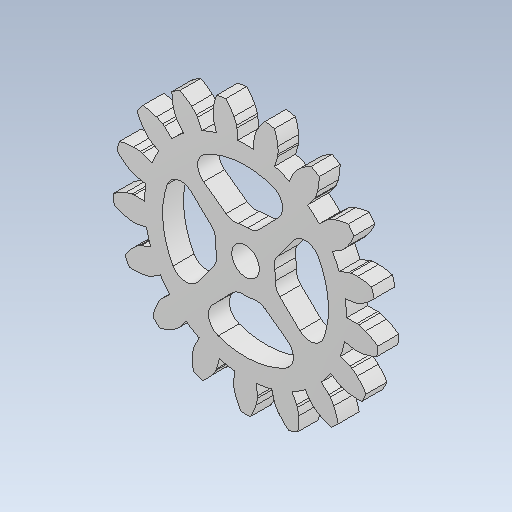
# Autodesk Inventor part: ｍ2歯数17ギアd3.99
Saved by Autodesk Inventor 2020.2 (Build 242310000, 310)
## iProperties
Created: 2020-03-11
Part Number: ｍ2歯数17ギアd3.99
Material: アルミニウム 2014-T4
Document SubType Name: Modeling
Designer: aoyam
Density: 2.8 g/cm^3
Appearance: サテン
Mass: 7.2939 g
Surface Area: 24.4586 cm^2
Volume: 2.60496 cm^3
Author: aoyam
Autodesk Inventor part; units mm, degrees
ref_plane "YZ Plane" through (0, 0, 0) normal (1, 0, 0) x (0, 1, 0)
ref_plane "XZ Plane" through (0, 0, 0) normal (0, 1, 0) x (-1, 0, 0)
ref_plane "XY Plane" through (0, 0, 0) normal (0, 0, 1) x (1, 0, 0)
sketch "スケッチ1" plane through (0, 0, 0) normal (0, 0, 1) x (1, 0, 0)
  arc A0 (3.6531, 18.9504) -> (3.5922, 18.6594) centre (5.3094, 18.4521) ccw
  arc A1 (4.0246, 19.8629) -> (3.6531, 18.9504) centre (8.2422, 17.6137) ccw
  arc A2 (5.1821, 21.5212) -> (4.0246, 19.8629) centre (11.4021, 15.9465) ccw
  arc A3 (1.1187, 18.6594) -> (1.0579, 18.9504) centre (-0.5985, 18.4521) ccw
  arc A4 (1.0579, 18.9504) -> (0.6864, 19.8629) centre (-3.5313, 17.6137) ccw
  arc A5 (0.6864, 19.8629) -> (-0.4711, 21.5212) centre (-6.6912, 15.9465) ccw
  arc A6 (3.478, 17.1891) -> (1.2329, 17.1891) centre (2.3555, 2.7326) ccw
  arc A7 (-0.4711, 21.5212) -> (-1.796, 21.2735) centre (2.3555, 2.7326) ccw
  line L0 (3.478, 17.1891) -> (3.5922, 18.6594)
  line L1 (1.2329, 17.1891) -> (1.1187, 18.6594)
  arc A8 (-4.5512, 17.1371) -> (-4.7131, 17.3865) centre (-6.0775, 16.3235) ccw
  line L2 (-3.9136, 15.8073) -> (-4.5512, 17.1371)
  arc A9 (-1.8201, 16.6184) -> (-3.9136, 15.8073) centre (2.3555, 2.7326) ccw
  line L3 (-1.8201, 16.6184) -> (-2.2447, 18.0307)
  arc A10 (-2.2931, 18.324) -> (-2.2447, 18.0307) centre (-0.5686, 18.4577) ccw
  arc A11 (-2.2763, 19.3091) -> (-2.2931, 18.324) centre (2.469, 18.7354) ccw
  arc A12 (-1.796, 21.2735) -> (-2.2763, 19.3091) centre (6.0178, 18.3222) ccw
  arc A13 (-4.7131, 17.3865) -> (-5.3891, 18.1031) centre (-8.5095, 14.4823) ccw
  arc A14 (-5.3891, 18.1031) -> (-7.0674, 19.2313) centre (-10.8537, 11.7862) ccw
  arc A15 (-7.0674, 19.2313) -> (-8.2134, 18.5218) centre (2.3555, 2.7326) ccw
  arc A16 (-9.2883, 13.6695) -> (-9.5294, 13.8435) centre (-10.4177, 12.3594) ccw
  line L4 (-8.2134, 12.6598) -> (-9.2883, 13.6695)
  arc A17 (-6.5542, 14.1723) -> (-8.2134, 12.6598) centre (2.3555, 2.7326) ccw
  line L5 (-6.5542, 14.1723) -> (-7.4604, 15.3358)
  arc A18 (-7.6115, 15.5919) -> (-7.4604, 15.3358) centre (-6.0517, 16.3395) ccw
  arc A19 (-7.9516, 16.5165) -> (-7.6115, 15.5919) centre (-3.3195, 17.6958) ccw
  arc A20 (-8.2134, 18.5218) -> (-7.9516, 16.5165) centre (0.1389, 18.5925) ccw
  arc A21 (-9.5294, 13.8435) -> (-10.4186, 14.2675) centre (-12.0203, 9.764) ccw
  arc A22 (-10.4186, 14.2675) -> (-12.3912, 14.7132) centre (-13.2323, 6.4031) ccw
  arc A23 (-12.3912, 14.7132) -> (-13.2034, 13.6376) centre (2.3555, 2.7326) ccw
  arc A24 (-12.4529, 8.7247) -> (-12.7406, 8.7999) centre (-13.0328, 7.0951) ccw
  line L6 (-11.0858, 8.1715) -> (-12.4529, 8.7247)
  arc A25 (-10.0851, 10.1813) -> (-11.0858, 8.1715) centre (2.3555, 2.7326) ccw
  line L7 (-10.0851, 10.1813) -> (-11.3504, 10.9389)
  arc A26 (-11.5838, 11.1231) -> (-11.3504, 10.9389) centre (-10.3994, 12.3836) ccw
  arc A27 (-12.2349, 11.8623) -> (-11.5838, 11.1231) centre (-8.3416, 14.6353) ccw
  arc A28 (-13.2034, 13.6376) -> (-12.2349, 11.8623) centre (-5.4407, 16.7208) ccw
  arc A29 (-12.7406, 8.7999) -> (-13.7229, 8.8741) centre (-13.5896, 4.0961) ccw
  arc A30 (-13.7229, 8.8741) -> (-15.7233, 8.5771) centre (-13.5056, 0.5243) ccw
  arc A31 (-15.7233, 8.5771) -> (-16.0921, 7.2807) centre (2.3555, 2.7326) ccw
  arc A32 (-13.6175, 2.9707) -> (-13.9129, 2.9369) centre (-13.5696, 1.2417) ccw
  line L8 (-12.1429, 2.9487) -> (-13.6175, 2.9707)
  arc A33 (-11.9358, 5.1842) -> (-12.1429, 2.9487) centre (2.3555, 2.7326) ccw
  line L9 (-11.9358, 5.1842) -> (-13.3893, 5.4336)
  arc A34 (-13.6735, 5.521) -> (-13.3893, 5.4336) centre (-13.0244, 7.1243) ccw
  arc A35 (-14.5477, 5.9752) -> (-13.6735, 5.521) centre (-11.9191, 9.9673) ccw
  arc A36 (-16.0921, 7.2807) -> (-14.5477, 5.9752) centre (-9.9674, 12.9599) ccw
  arc A37 (-13.9129, 2.9369) -> (-14.8558, 2.6512) centre (-13.0054, -1.756) ccw
  arc A38 (-14.8558, 2.6512) -> (-16.6138, 1.6516) centre (-11.6368, -5.0563) ccw
  arc A39 (-16.6138, 1.6516) -> (-16.4894, 0.3095) centre (2.3555, 2.7326) ccw
  arc A40 (-12.6249, -2.8155) -> (-12.8882, -2.9537) centre (-11.9556, -4.4104) ccw
  line L10 (-11.2419, -2.3033) -> (-12.6249, -2.8155)
  arc A41 (-11.8563, -0.1439) -> (-11.2419, -2.3033) centre (2.3555, 2.7326) ccw
  line L11 (-11.8563, -0.1439) -> (-13.3018, -0.4365)
  arc A42 (-13.5984, -0.4576) -> (-13.3018, -0.4365) centre (-13.5724, 1.2719) ccw
  arc A43 (-14.5777, -0.3499) -> (-13.5984, -0.4576) centre (-13.5686, 4.3222) ccw
  arc A44 (-16.4894, 0.3095) -> (-14.5777, -0.3499) centre (-12.8297, 7.8177) ccw
  arc A45 (-12.8882, -2.9537) -> (-13.6641, -3.5607) centre (-10.3466, -7.0019) ccw
  arc A46 (-13.6641, -3.5607) -> (-14.9423, -5.1278) centre (-7.8783, -9.5849) ccw
  arc A47 (-14.9423, -5.1278) -> (-14.3415, -6.3344) centre (2.3555, 2.7326) ccw
  arc A48 (-9.6091, -7.8524) -> (-9.8047, -8.0764) centre (-8.4088, -9.0978) ccw
  line L12 (-8.5046, -6.8752) -> (-9.6091, -7.8524)
  arc A49 (-9.8575, -5.0836) -> (-8.5046, -6.8752) centre (2.3555, 2.7326) ccw
  line L13 (-9.8575, -5.0836) -> (-11.0997, -5.8785)
  arc A50 (-11.3686, -6.0054) -> (-11.0997, -5.8785) centre (-11.9691, -4.3833) ccw
  arc A51 (-12.3207, -6.2587) -> (-11.3686, -6.0054) centre (-13.0675, -1.5376) ccw
  arc A52 (-14.3415, -6.3344) -> (-12.3207, -6.2587) centre (-13.6413, 1.9888) ccw
  arc A53 (-9.8047, -8.0764) -> (-10.3089, -8.9227) centre (-5.9724, -10.9331) ccw
  arc A54 (-10.3089, -8.9227) -> (-10.9347, -10.8457) centre (-2.7376, -12.45) ccw
  arc A55 (-10.9347, -10.8457) -> (-9.9386, -11.7538) centre (2.3555, 2.7326) ccw
  arc A56 (-4.9774, -11.4597) -> (-5.0789, -11.7392) centre (-3.4083, -12.1875) ccw
  line L14 (-4.3005, -10.1495) -> (-4.9774, -11.4597)
  arc A57 (-6.2093, -8.9676) -> (-4.3005, -10.1495) centre (2.3555, 2.7326) ccw
  line L15 (-6.2093, -8.9676) -> (-7.0804, -10.1576)
  arc A58 (-7.2854, -10.373) -> (-7.0804, -10.1576) centre (-8.4313, -9.0774) ccw
  arc A59 (-8.0816, -10.9532) -> (-7.2854, -10.373) centre (-10.4835, -6.8207) ccw
  arc A60 (-9.9386, -11.7538) -> (-8.0816, -10.9532) centre (-12.2924, -3.7397) ccw
  arc A61 (-5.0789, -11.7392) -> (-5.2433, -12.7106) centre (-0.4734, -13.0186) ccw
  arc A62 (-5.2433, -12.7106) -> (-5.1322, -14.7298) centre (3.0909, -13.2646) ccw
  arc A63 (-5.1322, -14.7298) -> (-3.8754, -15.2167) centre (2.3555, 2.7326) ccw
  arc A64 (0.6446, -13.1503) -> (0.651, -13.4476) centre (2.3707, -13.2621) ccw
  line L16 (0.8025, -11.684) -> (0.6446, -13.1503)
  arc A65 (-1.4043, -11.2715) -> (0.8025, -11.684) centre (2.3555, 2.7326) ccw
  line L17 (-1.4043, -11.2715) -> (-1.7867, -12.6958)
  arc A66 (-1.9001, -12.9707) -> (-1.7867, -12.6958) centre (-3.4366, -12.1765) ccw
  arc A67 (-2.4329, -13.7993) -> (-1.9001, -12.9707) centre (-6.1655, -10.8135) ccw
  arc A68 (-3.8754, -15.2167) -> (-2.4329, -13.7993) centre (-8.9652, -8.594) ccw
  arc A69 (0.651, -13.4476) -> (0.8485, -14.4127) centre (5.4076, -12.9769) ccw
  arc A70 (0.8485, -14.4127) -> (1.6815, -16.2555) centre (8.8201, -11.9187) ccw
  arc A71 (1.6815, -16.2555) -> (3.0294, -16.2555) centre (2.3555, 2.7326) ccw
  arc A72 (6.4977, -12.6958) -> (6.611, -12.9707) centre (8.1476, -12.1765) ccw
  line L18 (6.1153, -11.2715) -> (6.4977, -12.6958)
  arc A73 (3.9084, -11.684) -> (6.1153, -11.2715) centre (2.3555, 2.7326) ccw
  line L19 (3.9084, -11.684) -> (4.0663, -13.1503)
  arc A74 (4.06, -13.4476) -> (4.0663, -13.1503) centre (2.3403, -13.2621) ccw
  arc A75 (3.8625, -14.4127) -> (4.06, -13.4476) centre (-0.6966, -12.9769) ccw
  arc A76 (3.0294, -16.2555) -> (3.8625, -14.4127) centre (-4.1091, -11.9187) ccw
  arc A77 (6.611, -12.9707) -> (7.1439, -13.7993) centre (10.8764, -10.8135) ccw
  arc A78 (7.1439, -13.7993) -> (8.5863, -15.2167) centre (13.6762, -8.594) ccw
  arc A79 (8.5863, -15.2167) -> (9.8432, -14.7298) centre (2.3555, 2.7326) ccw
  arc A80 (11.7914, -10.1576) -> (11.9963, -10.373) centre (13.1422, -9.0774) ccw
  line L20 (10.9203, -8.9676) -> (11.7914, -10.1576)
  arc A81 (9.0114, -10.1495) -> (10.9203, -8.9676) centre (2.3555, 2.7326) ccw
  line L21 (9.0114, -10.1495) -> (9.6884, -11.4597)
  arc A82 (9.7898, -11.7392) -> (9.6884, -11.4597) centre (8.1193, -12.1875) ccw
  arc A83 (9.9543, -12.7106) -> (9.7898, -11.7392) centre (5.1844, -13.0186) ccw
  arc A84 (9.8432, -14.7298) -> (9.9543, -12.7106) centre (1.6201, -13.2646) ccw
  arc A85 (11.9963, -10.373) -> (12.7925, -10.9532) centre (15.1944, -6.8207) ccw
  arc A86 (12.7925, -10.9532) -> (14.6496, -11.7538) centre (17.0033, -3.7397) ccw
  arc A87 (14.6496, -11.7538) -> (15.6457, -10.8457) centre (2.3555, 2.7326) ccw
  arc A88 (15.8107, -5.8785) -> (16.0796, -6.0054) centre (16.6801, -4.3833) ccw
  line L22 (14.5685, -5.0836) -> (15.8107, -5.8785)
  arc A89 (13.2155, -6.8752) -> (14.5685, -5.0836) centre (2.3555, 2.7326) ccw
  line L23 (13.2155, -6.8752) -> (14.3201, -7.8524)
  arc A90 (14.5156, -8.0764) -> (14.3201, -7.8524) centre (13.1198, -9.0978) ccw
  arc A91 (15.0199, -8.9227) -> (14.5156, -8.0764) centre (10.6833, -10.9331) ccw
  arc A92 (15.6457, -10.8457) -> (15.0199, -8.9227) centre (7.4486, -12.45) ccw
  arc A93 (16.0796, -6.0054) -> (17.0316, -6.2587) centre (17.7785, -1.5376) ccw
  arc A94 (17.0316, -6.2587) -> (19.0525, -6.3344) centre (18.3522, 1.9888) ccw
  arc A95 (19.0525, -6.3344) -> (19.6533, -5.1278) centre (2.3555, 2.7326) ccw
  arc A96 (18.0128, -0.4365) -> (18.3093, -0.4576) centre (18.2833, 1.2719) ccw
  line L24 (16.5673, -0.1439) -> (18.0128, -0.4365)
  arc A97 (15.9529, -2.3033) -> (16.5673, -0.1439) centre (2.3555, 2.7326) ccw
  line L25 (15.9529, -2.3033) -> (17.3359, -2.8155)
  arc A98 (17.5991, -2.9537) -> (17.3359, -2.8155) centre (16.6665, -4.4104) ccw
  arc A99 (18.3751, -3.5607) -> (17.5991, -2.9537) centre (15.0576, -7.0019) ccw
  arc A100 (19.6533, -5.1278) -> (18.3751, -3.5607) centre (12.5892, -9.5849) ccw
  arc A101 (18.3093, -0.4576) -> (19.2886, -0.3499) centre (18.2795, 4.3222) ccw
  arc A102 (19.2886, -0.3499) -> (21.2003, 0.3095) centre (17.5407, 7.8177) ccw
  arc A103 (21.2003, 0.3095) -> (21.3247, 1.6516) centre (2.3555, 2.7326) ccw
  arc A104 (18.1003, 5.4336) -> (18.3844, 5.521) centre (17.7354, 7.1243) ccw
  line L26 (16.6467, 5.1842) -> (18.1003, 5.4336)
  arc A105 (16.8539, 2.9487) -> (16.6467, 5.1842) centre (2.3555, 2.7326) ccw
  line L27 (16.8539, 2.9487) -> (18.3285, 2.9707)
  arc A106 (18.6239, 2.9369) -> (18.3285, 2.9707) centre (18.2805, 1.2417) ccw
  arc A107 (19.5667, 2.6512) -> (18.6239, 2.9369) centre (17.7163, -1.756) ccw
  arc A108 (21.3247, 1.6516) -> (19.5667, 2.6512) centre (16.3477, -5.0563) ccw
  arc A109 (18.3844, 5.521) -> (19.2587, 5.9752) centre (16.63, 9.9673) ccw
  arc A110 (19.2587, 5.9752) -> (20.8031, 7.2807) centre (14.6783, 12.9599) ccw
  arc A111 (20.8031, 7.2807) -> (20.4342, 8.5771) centre (2.3555, 2.7326) ccw
  arc A112 (16.0613, 10.9389) -> (16.2947, 11.1231) centre (15.1103, 12.3836) ccw
  line L28 (14.796, 10.1813) -> (16.0613, 10.9389)
  arc A113 (15.7968, 8.1715) -> (14.796, 10.1813) centre (2.3555, 2.7326) ccw
  line L29 (15.7968, 8.1715) -> (17.1638, 8.7247)
  arc A114 (17.4515, 8.7999) -> (17.1638, 8.7247) centre (17.7437, 7.0951) ccw
  arc A115 (18.4339, 8.8741) -> (17.4515, 8.7999) centre (18.3005, 4.0961) ccw
  arc A116 (20.4342, 8.5771) -> (18.4339, 8.8741) centre (18.2165, 0.5243) ccw
  arc A117 (16.2947, 11.1231) -> (16.9459, 11.8623) centre (13.0526, 14.6353) ccw
  arc A118 (16.9459, 11.8623) -> (17.9144, 13.6376) centre (10.1516, 16.7208) ccw
  arc A119 (17.9144, 13.6376) -> (17.1021, 14.7132) centre (2.3555, 2.7326) ccw
  arc A120 (12.1714, 15.3358) -> (12.3224, 15.5919) centre (10.7627, 16.3395) ccw
  line L30 (11.2652, 14.1723) -> (12.1714, 15.3358)
  arc A121 (12.9243, 12.6598) -> (11.2652, 14.1723) centre (2.3555, 2.7326) ccw
  line L31 (12.9243, 12.6598) -> (13.9993, 13.6695)
  arc A122 (14.2403, 13.8435) -> (13.9993, 13.6695) centre (15.1286, 12.3594) ccw
  arc A123 (15.1296, 14.2675) -> (14.2403, 13.8435) centre (16.7312, 9.764) ccw
  arc A124 (17.1021, 14.7132) -> (15.1296, 14.2675) centre (17.9432, 6.4031) ccw
  arc A125 (12.3224, 15.5919) -> (12.6626, 16.5165) centre (8.0305, 17.6958) ccw
  arc A126 (12.6626, 16.5165) -> (12.9244, 18.5218) centre (4.5721, 18.5925) ccw
  arc A127 (12.9244, 18.5218) -> (11.7784, 19.2313) centre (2.3555, 2.7326) ccw
  arc A128 (6.9557, 18.0307) -> (7.0041, 18.324) centre (5.2796, 18.4577) ccw
  line L32 (6.531, 16.6184) -> (6.9557, 18.0307)
  arc A129 (8.6245, 15.8073) -> (6.531, 16.6184) centre (2.3555, 2.7326) ccw
  line L33 (8.6245, 15.8073) -> (9.2621, 17.1371)
  arc A130 (9.424, 17.3865) -> (9.2621, 17.1371) centre (10.7885, 16.3235) ccw
  arc A131 (10.1001, 18.1031) -> (9.424, 17.3865) centre (13.2204, 14.4823) ccw
  arc A132 (11.7784, 19.2313) -> (10.1001, 18.1031) centre (15.5647, 11.7862) ccw
  arc A133 (7.0041, 18.324) -> (6.9872, 19.3091) centre (2.2419, 18.7354) ccw
  arc A134 (6.9872, 19.3091) -> (6.507, 21.2735) centre (-1.3069, 18.3222) ccw
  arc A135 (6.507, 21.2735) -> (5.1821, 21.5212) centre (2.3555, 2.7326) ccw
  circle A136 centre (2.3555, 2.7326) radius 1.995
  circle A137 centre (2.3555, 2.7326) radius 14.5
  circle A138 centre (2.3555, 2.7326) radius 11.9
  circle A139 centre (2.3555, 2.7326) radius 4.295
  line L34 (2.3555, 2.7326) -> (10.0109, 11.8433)
  line L35 (10.8895, 11.026) -> (6.2096, 4.628)
  line L36 (9.0544, 12.5679) -> (3.5584, 6.8557)
  line L37 (-7.4799, 9.4315) -> (-1.7676, 3.9355)
  line L38 (-5.9379, 11.2666) -> (0.4601, 6.5867)
  line L39 (-4.3435, -7.1028) -> (1.1525, -1.3905)
  line L40 (-6.1786, -5.5608) -> (-1.4987, 0.8372)
  line L41 (12.1908, -3.9664) -> (6.4786, 1.5296)
  line L42 (10.6488, -5.8015) -> (4.2508, -1.1216)
  point P0 (0, 0)
  point P1 (-4.5512, 17.1371)
  point P2 (-4.7131, 17.3865)
  point P3 (-5.3891, 18.1031)
  point P4 (-7.0674, 19.2313)
  point P5 (-8.2134, 18.5218)
  point P6 (-7.9516, 16.5165)
  point P7 (-7.6115, 15.5919)
  point P8 (-7.4604, 15.3358)
  point P9 (-6.5542, 14.1723)
  point P10 (-9.5294, 13.8435)
  point P11 (-10.4186, 14.2675)
  point P12 (-12.3912, 14.7132)
  point P13 (-13.2034, 13.6376)
  point P14 (-11.5838, 11.1231)
  point P15 (-11.3504, 10.9389)
  point P16 (-10.0851, 10.1813)
  point P17 (-11.0858, 8.1715)
  point P18 (-12.4529, 8.7247)
  point P19 (-12.7406, 8.7999)
  point P20 (-13.7229, 8.8741)
  point P21 (-15.7233, 8.5771)
  point P22 (-16.0921, 7.2807)
  point P23 (-14.5477, 5.9752)
  point P24 (-13.6735, 5.521)
  point P25 (-13.3893, 5.4336)
  point P26 (-11.9358, 5.1842)
  point P27 (-12.1429, 2.9487)
  point P28 (-13.6175, 2.9707)
  point P29 (-13.9129, 2.9369)
  point P30 (-14.8558, 2.6512)
  point P31 (-16.6138, 1.6516)
  point P32 (-16.4894, 0.3095)
  point P33 (-14.5777, -0.3499)
  point P34 (-13.5984, -0.4576)
  point P35 (-12.8882, -2.9537)
  point P36 (-13.6641, -3.5607)
  point P37 (-14.9423, -5.1278)
  point P38 (-14.3415, -6.3344)
  point P39 (-12.3207, -6.2587)
  point P40 (-11.3686, -6.0054)
  point P41 (-11.0997, -5.8785)
  point P42 (-9.8575, -5.0836)
  point P43 (-10.3089, -8.9227)
  point P44 (-10.9347, -10.8457)
  point P45 (-9.9386, -11.7538)
  point P46 (-8.0816, -10.9532)
  point P47 (-7.2854, -10.373)
  point P48 (-7.0804, -10.1576)
  point P49 (-5.0789, -11.7392)
  point P50 (-5.2433, -12.7106)
  point P51 (-5.1322, -14.7298)
  point P52 (-3.8754, -15.2167)
  point P53 (-2.4329, -13.7993)
  point P54 (-1.9001, -12.9707)
  point P55 (-1.7867, -12.6958)
  point P56 (0.651, -13.4476)
  point P57 (0.8485, -14.4127)
  point P58 (1.6815, -16.2555)
  point P59 (3.0294, -16.2555)
  point P60 (3.8625, -14.4127)
  point P61 (4.06, -13.4476)
  point P62 (4.0663, -13.1503)
  point P63 (3.9084, -11.684)
  point P64 (6.1153, -11.2715)
  point P65 (6.4977, -12.6958)
  point P66 (6.611, -12.9707)
  point P67 (7.1439, -13.7993)
  point P68 (8.5863, -15.2167)
  point P69 (9.8432, -14.7298)
  point P70 (9.9543, -12.7106)
  point P71 (9.7898, -11.7392)
  point P72 (9.6884, -11.4597)
  point P73 (9.0114, -10.1495)
  point P74 (11.9963, -10.373)
  point P75 (12.7925, -10.9532)
  point P76 (14.6496, -11.7538)
  point P77 (15.6457, -10.8457)
  point P78 (15.0199, -8.9227)
  point P79 (14.5156, -8.0764)
  point P80 (14.3201, -7.8524)
  point P81 (13.2155, -6.8752)
  point P82 (16.0796, -6.0054)
  point P83 (17.0316, -6.2587)
  point P84 (19.0525, -6.3344)
  point P85 (19.6533, -5.1278)
  point P86 (18.3751, -3.5607)
  point P87 (17.5991, -2.9537)
  point P88 (18.0128, -0.4365)
  point P89 (18.3093, -0.4576)
  point P90 (19.2886, -0.3499)
  point P91 (21.2003, 0.3095)
  point P92 (21.3247, 1.6516)
  point P93 (19.5667, 2.6512)
  point P94 (18.6239, 2.9369)
  point P95 (18.3285, 2.9707)
  point P96 (18.1003, 5.4336)
  point P97 (18.3844, 5.521)
  point P98 (19.2587, 5.9752)
  point P99 (20.8031, 7.2807)
  point P100 (20.4342, 8.5771)
  point P101 (18.4339, 8.8741)
  point P102 (17.4515, 8.7999)
  point P103 (17.1638, 8.7247)
  point P104 (14.796, 10.1813)
  point P105 (16.2947, 11.1231)
  point P106 (16.9459, 11.8623)
  point P107 (17.9144, 13.6376)
  point P108 (17.1021, 14.7132)
  point P109 (15.1296, 14.2675)
  point P110 (14.2403, 13.8435)
  point P111 (12.3224, 15.5919)
  point P112 (12.6626, 16.5165)
  point P113 (12.9244, 18.5218)
  point P114 (11.7784, 19.2313)
  point P115 (10.1001, 18.1031)
  point P116 (9.424, 17.3865)
  point P117 (6.9557, 18.0307)
  point P118 (7.0041, 18.324)
  point P119 (6.9872, 19.3091)
  point P120 (6.507, 21.2735)
  point P121 (5.1821, 21.5212)
  point P122 (4.0246, 19.8629)
  point P123 (3.6531, 18.9504)
  point P124 (3.5922, 18.6594)
  point P125 (3.478, 17.1891)
  point P126 (1.2329, 17.1891)
  point P127 (1.1187, 18.6594)
  point P128 (1.0579, 18.9504)
  point P129 (0.6864, 19.8629)
  point P130 (-0.4711, 21.5212)
  point P131 (-1.796, 21.2735)
  point P132 (-2.2763, 19.3091)
  point P133 (-2.2931, 18.324)
  point P134 (-2.2447, 18.0307)
  point P135 (3.5584, 6.8557)
  point P136 (0.4601, 6.5867)
  point P137 (9.0544, 12.5679)
  point P138 (12.1908, -3.9664)
  point P139 (6.4786, 1.5296)
  point P140 (1.1525, -1.3905)
  point P141 (4.2508, -1.1216)
  point P142 (10.6488, -5.8015)
  point P143 (-4.3435, -7.1028)
  point P144 (-1.7676, 3.9355)
  point P145 (-1.4987, 0.8372)
  point P146 (-7.4799, 9.4315)
  dimension "d2" = 360
  dimension "d4" = 3.99
  dimension "d7" = 29
  dimension "d8" = 2.6
  dimension "d9" = 2.3
  dimension "d10" = 1.2
  dimension "d13" = 360
  constraints: 274 point on circle, 139 centre point, 86 end point, 5 coincident, 2 symmetric about line, 1 concentric, 675 other
  measures "d4" diameter of A136
  measures "d7" diameter of A137
  measures "d8" radial gap between concentric circles of A137 A138
  measures "d10" distance of L35.start L34.end
extrude "押し出し1" add sketch "スケッチ1" along normal blind 3 contours A1 A2 A135 A134 A133 A128 L32 A137 L0 A0 | A137 A129 A121 A113 A105 A97 A89 A81 A73 A65 A57 A49 A41 A33 A25 A17 A9 A6 | A137 L3 A10 A11 A12 A7 A5 A4 A3 L1 | L33 A130 A131 A132 A127 A126 A125 A120 L30 A137 | A137 L5 A18 A19 A20 A15 A14 A13 A8 L2 | L31 A122 A123 A124 A119 A118 A117 A112 L28 A137 | A137 L7 A26 A27 A28 A23 A22 A21 A16 L4 | L29 A114 A115 A116 A111 A110 A109 A104 L26 A137 | A137 L9 A34 A35 A36 A31 A30 A29 A24 L6 | L27 A106 A107 A108 A103 A102 A101 A96 L24 A137 | A137 L11 A42 A43 A44 A39 A38 A37 A32 L8 | A137 L13 A50 A51 A52 A47 A46 A45 A40 L10 | L25 A98 A99 A100 A95 A94 A93 A88 L22 A137 | A137 L15 A58 A59 A60 A55 A54 A53 A48 L12 | L23 A90 A91 A92 A87 A86 A85 A80 L20 A137 | A137 L17 A66 A67 A68 A63 A62 A61 A56 L14 | L21 A82 A83 A84 A79 A78 A77 A72 L18 A137 | A137 L19 A74 A75 A76 A71 A70 A69 A64 L16 | A139 | A139 L36 A138 L34 | L34 A138 L35 A139 | A139 L37 A138 L38 | L41 A138 L42 A139 | A139 L39 A138 L40
fillet "フィレット1" radius 2.1 16 edges at (0.4601, 6.5867, 1.5) (3.5584, 6.8557, 1.5) (-5.9379, 11.2666, 1.5) (9.0544, 12.5679, 1.5) (-7.4799, 9.4315, 1.5) (-1.7676, 3.9355, 1.5) (-1.4987, 0.8372, 1.5) (-6.1786, -5.5608, 1.5) (-4.3435, -7.1028, 1.5) (4.2508, -1.1216, 1.5) (1.1525, -1.3905, 1.5) (10.6488, -5.8015, 1.5) (12.1908, -3.9664, 1.5) (6.4786, 1.5296, 1.5) (6.2096, 4.628, 1.5) (10.8895, 11.026, 1.5)
